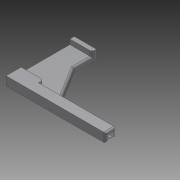
# Autodesk Inventor part: Tirador
Saved by Autodesk Inventor 2011 (Build 150239000, 239)
## iProperties
Created: 2014-08-04
Part Number: Tirador
Material: Por defecto
Document SubType Name: Chapa
Designer: amatiasq
Density: 1 g/cm^3
Sheet Metal Rule: Por defecto_mm
Author: amatiasq
Autodesk Inventor part; units mm, degrees
ref_plane "YZ Plane" through (0, 0, 0) normal (1, 0, 0) x (0, 1, 0)
ref_plane "XZ Plane" through (0, 0, 0) normal (0, 1, 0) x (-1, 0, 0)
ref_plane "XY Plane" through (0, 0, 0) normal (0, 0, 1) x (1, 0, 0)
sketch "Boceto1" plane through (0, 0, 0) normal (0, 0, 1) x (1, 0, 0)
  line L0 (0, 0) -> (0, 30.8)
  line L1 (0, 30.8) -> (10, 30.8)
  line L2 (10, 30.8) -> (10, 20.8)
  line L3 (0, 0) -> (45, 0)
  line L4 (45, 0) -> (45, 4.6)
  line L5 (45, 4.6) -> (20, 4.6)
  line L6 (20, 4.6) -> (10, 20.8)
  dimension "d0" = 30.8
  dimension "d1" = 10
  dimension "d2" = 10
  dimension "d3" = 45
  dimension "d4" = 4.6
  dimension "d5" = 25
  constraints: 14 end point, 3 perpendicular, 2 parallel, 1 vertical
  measures "d0" distance of L0.start L0.end
  measures "d1" distance of L0.end L1.end
  measures "d2" distance of L1.end L2.end
  measures "d3" distance of L0.start L3.end
  measures "d4" distance of L3.end L4.end
  measures "d5" distance of L4.end L5.end
extrude "Extrusión1" add sketch "Boceto1" along normal blind 1.8
sketch "Boceto2" plane through (0, 0, 1.8) normal (0, 0, 1) x (1, 0, 0)
  line L0 (0, 0) -> (0, 30.8) projected
  line L1 (45, 0) -> (0, 0) projected
  line L2 (45, 4.6) -> (45, 0) projected
  line L3 (20, 4.6) -> (45, 4.6) projected
  line L4 (10, 30.8) -> (10, 20.8) projected
  line L5 (20, 4.6) -> (10, 4.6)
  line L6 (0, 6.8) -> (10, 6.8)
  line L7 (10, 6.8) -> (10, 4.6)
  line L8 (0, 30.8) -> (10, 30.8)
  line L9 (10, 30.8) -> (10, 28.8)
  line L10 (10, 28.8) -> (0, 28.8)
  line L11 (0, 28.8) -> (0, 30.8)
  dimension "d8" = 10
  dimension "d9" = 10
  dimension "d14" = 6.8
  dimension "d18" = 2
  constraints: 14 end point, 3 parallel, 2 perpendicular, 2 point on line, 1 horizontal
  measures "d8" distance of L3.start L5.end
  measures "d9" distance of L6.start L6.end
  measures "d14" distance of L0.start L6.start
  measures "d18" distance of L8.end L9.end
extrude "Extrusión2" add sketch "Boceto2" along normal blind 2.2
fillet "Empalme1" radius 1 4 edges at (45, 0, 2) (45, 2.3, 0) (45, 4.6, 2) (45, 2.3, 4)
fillet "Empalme2" radius 1 4 edges at (10, 6.8, 2.9) (10, 28.8, 2.9) (15, 12.7, 1.8) (10, 24.8, 1.8)
sketch "Boceto3" plane through (45, 1, 3) normal (1, 0, 0) x (0, 0, -1)
  line L0 (2, 0) -> (0, 0) projected
  line L1 (2, 2.6) -> (2, 0) projected
  point P0 (3, -1)
  point P1 (1, 1)
  dimension "d20" = 1
  dimension "d21" = 1
  measures "d20" distance from line of L0 point (1, 1)
  measures "d21" distance from line of L1 point (1, 1)
hole "Hole1" at (45, 2, 2) direction (-1, 0, 0) diameter 1 depth 3
equation "\"Radio_pliegue\" = Grosor"
equation "\"Anchura_desahogo_plegado\" = Grosor"
equation "\"Profundidad_desahogo_plegado\" = 0.5 * Grosor"
equation "\"Tamaño_destalonado\" = 4 * Grosor"
equation "\"Remanente_mínimo\" = 2 * Grosor"
equation "\"Radiodetransición\" = Radio_pliegue"
equation "\"Tamaño_de_radio_de_Jacobi\" = Radio_pliegue"
equation "\"TamañoSeparación\" = Grosor"
equation "\"Grosor\" = 0.5"
